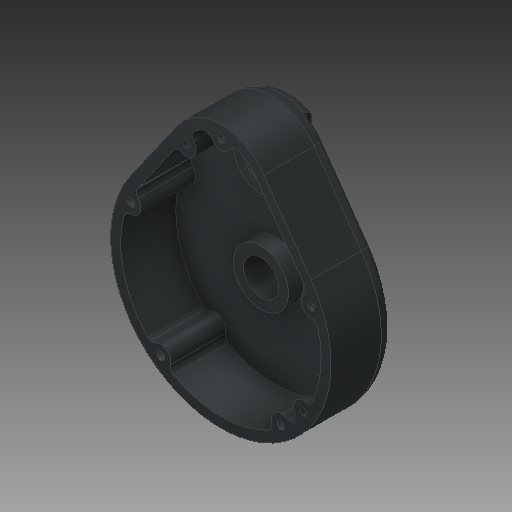
# Autodesk Inventor part: Caja1
Saved by Autodesk Inventor 2020 (Build 240168000, 168)
## iProperties
Created: 2016-04-19
Part Number: Caja1
Material: Iron, Cast
Document SubType Name: Modeling
Designer: Jorge
Density: 7.15 g/cm^3
Appearance: Iron Gray
Mass: 1669.68 g
Surface Area: 742.961 cm^2
Volume: 233.522 cm^3
Author: Jorge
Autodesk Inventor part; units mm, degrees
ref_plane "YZ Plane" through (0, 0, 0) normal (1, 0, 0) x (0, 1, 0)
ref_plane "XZ Plane" through (0, 0, 0) normal (0, 1, 0) x (-1, 0, 0)
ref_plane "XY Plane" through (0, 0, 0) normal (0, 0, 1) x (1, 0, 0)
sketch "Sketch1" plane through (0, 0, 0) normal (0, 0, 1) x (1, 0, 0)
  line L0 (57.148, 40.1638) -> (27.2752, 82.6691)
  arc A0 (27.2752, 82.6691) -> (-27.2752, 82.6691) centre (0, 63.5) ccw
  line L1 (-27.2752, 82.6691) -> (-57.148, 40.1638)
  arc A1 (-57.148, 40.1638) -> (57.148, 40.1638) centre (0, 0) ccw
  line L2 (-97.79, 0) -> (97.79, 0) construction
  circle A2 centre (0, 0) radius 11.1125
  circle A3 centre (0, 63.5) radius 11.1125
  line L3 (0, -103.1875) -> (0, 130.175) construction
  dimension "d21" = 33.3375
  dimension "d23" = 69.85
  dimension "d24" = 63.5
  dimension "d25" = 22.225
  dimension "d27" = 0
  constraints: 4 centre point, 4 end point, 4 point on circle, 4 tangent, 3 coincident, 1 equal radius
  measures "d21" radius of A0
  measures "d23" radius of A1
  measures "d24" distance of point (0, 0) A0.centre
  measures "d25" diameter of A2
  measures "d27" distance from line of L3 A0.centre
extrude "Extrusion2" add sketch "Sketch1" against normal blind 41.275
sketch "Sketch3" plane through (0, 0, 0) normal (0, 0, 1) x (1, 0, 0)
  circle A0 centre (0, 63.5) radius 11.1125 construction
  line L0 (-51.9527, 36.5125) -> (-29.9545, 67.8132)
  line L1 (22.0799, 79.0178) -> (51.9527, 36.5125)
  arc A1 (-57.4985, 19.0596) -> (-52.6772, 29.9074) centre (-57.15, 25.4) ccw
  arc A2 (-25.0533, 68.989) -> (-17.4133, 78.9063) centre (-22.0799, 74.5998) ccw
  arc A3 (-5.5475, 85.81) -> (5.5475, 85.81) centre (0, 88.9) ccw
  arc A4 (-32.0833, -51.2429) -> (-41.5727, -43.8962) centre (-38.1, -49.2125) ccw
  arc A5 (53.5354, -28.682) -> (47.0078, -38.3187) centre (52.3748, -34.925) ccw
  line L2 (0, -103.1875) -> (0, 130.175) construction
  line L3 (-97.79, 0) -> (97.79, 0) construction
  arc A6 (-51.9527, 36.5125) -> (-53.1847, 34.6935) centre (0, 0) ccw
  arc A7 (-61.3911, 16.2291) -> (-46.4429, -43.3048) centre (0, 0) ccw
  arc A8 (52.6772, 29.9074) -> (57.4985, 19.0596) centre (57.15, 25.4) ccw
  arc A9 (41.489, -43.8425) -> (32.0833, -51.2429) centre (38.1, -49.2125) ccw
  arc A10 (57.6934, -26.5278) -> (61.3911, 16.2291) centre (0, 0) ccw
  arc A11 (53.1847, 34.6935) -> (51.9527, 36.5125) centre (0, 0) ccw
  arc A12 (22.0799, 79.0178) -> (11.7884, 87.7767) centre (0, 63.5) ccw
  arc A13 (-11.7884, 87.7767) -> (-17.0156, 84.4474) centre (0, 63.5) ccw
  arc A14 (-25.0533, 68.989) -> (-29.9545, 67.8132) centre (-26.8374, 65.6225) ccw
  arc A15 (-53.1847, 34.6935) -> (-52.6772, 29.9074) centre (-49.9936, 32.6119) ccw
  arc A16 (-57.4985, 19.0596) -> (-61.3911, 16.2291) centre (-57.7076, 15.2553) ccw
  arc A17 (-46.4429, -43.3048) -> (-41.5727, -43.8962) centre (-43.6564, -40.7065) ccw
  arc A18 (-32.0833, -51.2429) -> (-30.2908, -55.8097) centre (-28.4734, -52.4611) ccw
  arc A19 (30.2908, -55.8097) -> (32.0833, -51.2429) centre (28.4734, -52.4611) ccw
  arc A20 (53.5354, -28.682) -> (57.6934, -26.5278) centre (54.2318, -24.9361) ccw
  arc A21 (61.3911, 16.2291) -> (57.4985, 19.0596) centre (57.7076, 15.2553) ccw
  arc A22 (52.6772, 29.9074) -> (53.1847, 34.6935) centre (49.9936, 32.6119) ccw
  arc A23 (-17.0156, 84.4474) -> (-17.4133, 78.9063) centre (-14.6134, 81.4901) ccw
  arc A24 (-5.5475, 85.81) -> (-11.7884, 87.7767) centre (-9.7081, 83.4926) ccw
  arc A25 (11.7884, 87.7767) -> (5.5475, 85.81) centre (9.7081, 83.4926) ccw
  arc A26 (41.489, -43.8425) -> (47.0078, -38.3187) centre (43.625, -40.4578) ccw
  arc A27 (-30.2908, -55.8097) -> (30.2908, -55.8097) centre (0, 0) ccw
  point P0 (-27.5047, 71.2991)
  dimension "d34" = 49.2125
  dimension "d35" = 25.4
  dimension "d36" = 57.15
  dimension "d37" = 38.1
  dimension "d38" = 74.5998
  dimension "d39" = 88.9
  dimension "d40" = 0
  dimension "d41" = 52.3748
  dimension "d42" = 34.925
  dimension "d43" = 6.35
  dimension "d45" = 26.9875
  dimension "d46" = 3.81
  dimension "d47" = 4.7625
  dimension "d111" = 4.0023
  constraints: 55 point on circle, 28 tangent, 27 centre point, 13 equal radius, 4 end point, 2 coincident, 2 symmetric about line, 1 point on line, 2 other
  measures "d34" distance from line of A4.centre L3
  measures "d35" distance from line of A1.centre L3
  measures "d36" distance from line of L2 A1.centre
  measures "d37" distance from line of L2 A4.centre
  measures "d38" distance from line of A2.centre L3
  measures "d39" distance from line of L3 A3.centre
  measures "d40" distance from line of L2 A3.centre
  measures "d41" distance from line of A5.centre L2
  measures "d42" distance from line of A5.centre L3
  measures "d43" radius of A3
  measures "d45" radius of A13
  measures "d46" radius of A14
  measures "d47" radius of A24
  measures "d111" radius of A26
extrude "Extrusion3" cut sketch "Sketch3" against normal blind 34.925
sketch "Sketch4" plane through (0, 0, -34.925) normal (0, 0, 1) x (1, 0, 0)
  circle A0 centre (0, 63.5) radius 11.1125 projected
  circle A1 centre (0, 0) radius 11.1125 projected
  arc A2 (-7.6278, 79.2085) -> (7.6278, 79.2085) centre (0, 63.5) ccw
  circle A3 centre (0, 0) radius 17.4625
  arc A4 (-5.5475, 85.81) -> (5.5475, 85.81) centre (0, 88.9) ccw projected
  arc A5 (-5.5475, 85.81) -> (5.5475, 85.81) centre (0, 88.9) ccw
  arc A6 (-7.6278, 79.2085) -> (-5.5475, 85.81) centre (-9.7081, 83.4926) ccw
  arc A7 (5.5475, 85.81) -> (7.6278, 79.2085) centre (9.7081, 83.4926) ccw
  arc A8 (-5.5475, 85.81) -> (5.5475, 85.81) centre (0, 88.9) ccw projected
  dimension "d48" = 34.925
  dimension "d51" = 4.7625
  constraints: 10 point on circle, 5 centre point, 4 tangent, 2 coincident, 2 equal radius, 1 concentric
  measures "d48" diameter of A3
  measures "d51" radius of A6
extrude "Extrusion4" add sketch "Sketch4" along normal blind 9.5631
sketch "Sketch7" plane through (0, 0, 0) normal (0, 1, 0) x (-1, 0, 0)
  line L0 (14.2875, -41.275) -> (-14.2875, -41.275)
  line L1 (-14.2875, -41.275) -> (-14.2875, -42.8625)
  line L2 (14.2875, -42.8625) -> (14.2875, -41.275)
  line L3 (0, -53.7345) -> (0, 8.9558) construction
  line L4 (-27.2752, -41.275) -> (27.2752, -41.275) construction
  arc A0 (7.9375, -44.45) -> (6.35, -44.45) centre (7.1438, -44.45) ccw
  line L5 (7.9375, -44.45) -> (12.7, -44.45)
  arc A1 (0, -44.45) -> (-1.5875, -44.45) centre (-0.7937, -44.45) ccw
  arc A2 (-7.9375, -44.45) -> (-9.525, -44.45) centre (-8.7312, -44.45) ccw
  line L6 (0, -44.45) -> (6.35, -44.45)
  line L7 (-12.7, -44.45) -> (-9.525, -44.45)
  line L8 (-7.9375, -44.45) -> (-1.5875, -44.45)
  arc A3 (-14.2875, -42.8625) -> (-12.7, -44.45) centre (-12.7, -42.8625) ccw
  arc A4 (12.7, -44.45) -> (14.2875, -42.8625) centre (12.7, -42.8625) ccw
  point P0 (0, 0)
  point P1 (-14.2875, -44.45)
  point P2 (14.2875, -44.45)
  dimension "d66" = 28.575
  dimension "d67" = 14.2875
  dimension "d69" = 0
  dimension "d70" = 7.1437
  dimension "d71" = 0.7937
  dimension "d74" = 7.9375
  dimension "d96" = 1.5875
  constraints: 14 end point, 10 point on circle, 5 centre point, 5 parallel, 4 point on line, 4 tangent, 2 horizontal, 1 equal radius, 1 perpendicular, 8 other
  measures "d66" distance between parallel lines of L1 L2
  measures "d67" distance between parallel lines of L3 L2
  measures "d69" distance between parallel lines of L4 L0
  measures "d70" distance from line of A0.centre L2
  measures "d71" radius of A0
  measures "d74" distance of A0.centre A1.centre
  measures "d96" radius of A3
extrude "Extrusion5" add sketch "Sketch7" along normal blind 96.8502 and the other way blind 69.85
sketch "Sketch8" plane through (0, 0, 0) normal (1, 0, 0) x (0, 1, 0)
  line L0 (0, -54.3176) -> (0, 9.0529) construction
  line L1 (40.1637, -41.275) -> (40.1637, -41.275) construction
  line L2 (96.8502, -43.6563) -> (-69.85, -43.6563) construction
  line L3 (-66.675, -41.275) -> (-78.3505, -41.275)
  line L4 (-69.85, -41.275) -> (-68.3732, -41.275) projected
  line L5 (-66.675, -41.275) -> (-66.675, -42.8625) construction
  line L6 (-78.3505, -41.275) -> (-78.3505, -44.5144)
  line L7 (-78.3505, -44.5144) -> (-61.1391, -44.5144)
  arc A0 (-66.675, -41.275) -> (-61.1391, -44.5144) centre (-61.1391, -38.1644) ccw
  point P0 (0, 0)
  point P1 (-65.0868, -44.5144)
  dimension "d84" = 0
  dimension "d87" = 66.675
  dimension "d106" = 6.35
  dimension "d107" = 3.2394
  constraints: 8 end point, 2 horizontal, 2 point on circle, 2 vertical, 1 centre point, 1 horizontal alignment, 1 point on line, 1 tangent
  measures "d84" distance between parallel lines of L4 L3
  measures "d87" distance between parallel lines of L5 L0
  measures "d106" radius of A0
  measures "d107" distance between parallel lines of L3 L7
revolve "Revolution1" cut sketch "Sketch8" angle 180 mid plane about axis through (0, 0, -10) along (0, 0, 1)
sketch "Sketch9" plane through (0, 0, 0) normal (1, 0, 0) x (0, 1, 0)
  line L0 (96.8502, -43.6563) -> (-63.7315, -43.6563) construction
  line L1 (93.6207, -41.275) -> (96.8502, -41.275) construction
  line L2 (82.6691, -41.275) -> (82.6691, -41.275) construction
  line L3 (93.6625, -41.275) -> (109.3342, -41.275)
  line L4 (63.5, 9.0374) -> (63.5, -54.2241) construction
  line L5 (109.3342, -44.45) -> (88.1632, -44.45)
  line L6 (93.6625, -41.275) -> (93.6625, -42.8625) construction
  line L7 (109.3342, -44.45) -> (109.3342, -41.275)
  arc A0 (88.1632, -44.45) -> (93.6625, -41.275) centre (88.1632, -38.1) ccw
  point P0 (0, 0)
  point P1 (92.075, -44.45)
  dimension "d98" = 30.1625
  dimension "d108" = 6.35
  dimension "d109" = 3.175
  constraints: 8 end point, 2 point on circle, 2 vertical, 1 centre point, 1 horizontal, 1 horizontal alignment, 1 parallel, 1 point on line, 1 tangent
  measures "d98" distance between parallel lines of L6 L4
  measures "d108" radius of A0
  measures "d109" distance from line of L3 L5.start
revolve "Revolution2" cut sketch "Sketch9" angle 90 mid plane about axis through (0, 63.5, 0) along (0, 0, -1)
sketch "Sketch10" plane through (0, 0, 0) normal (1, 0, 0) x (0, 1, 0)
  line L0 (-69.85, -44.45) -> (96.8502, -44.45) projected
  line L1 (-69.85, -41.275) -> (40.1638, -41.275) construction
  line L2 (-14.2875, -41.275) -> (-14.2875, -41.275)
  line L3 (0, -63.0631) -> (0, 10.5105) construction
  line L4 (-14.2875, -41.275) -> (0, -41.275)
  line L5 (11.1125, -41.275) -> (-11.1125, -41.275) projected
  line L6 (-19.7868, -44.45) -> (0, -44.45)
  line L7 (-69.85, -44.45) -> (96.8502, -44.45) projected
  line L8 (0, -44.45) -> (0, -41.275)
  line L9 (-69.85, -44.45) -> (96.8502, -44.45) projected
  arc A0 (-19.7868, -44.45) -> (-14.2875, -41.275) centre (-19.7868, -38.1) ccw
  line L10 (-14.2875, -41.275) -> (-14.2875, -52.5526) construction
  point P0 (0, 0)
  point P1 (-11.2175, -44.45)
  point P2 (-64.601, -44.45)
  point P3 (90.9504, -44.45)
  point P4 (-15.875, -44.45)
  point P5 (149.2752, -44.45)
  point P6 (-63.8357, -44.45)
  point P7 (89.0977, -44.45)
  point P8 (-61.531, -44.45)
  point P9 (-60.7271, -44.45)
  point P10 (84.642, -44.45)
  dimension "d103" = 6.35
  dimension "d104" = 14.2875
  constraints: 10 end point, 4 point on line, 2 point on circle, 1 centre point, 1 midpoint, 1 perpendicular, 1 tangent, 1 vertical, 3 other
  measures "d103" radius of A0
  measures "d104" distance between parallel lines of L3 L10
revolve "Revolution3" cut sketch "Sketch10" angle 360 about axis through (0, 0, -10) along (0, 0, 1)
sketch "Sketch11" plane through (0, 0, 0) normal (1, 0, 0) x (0, 1, 0)
  line L0 (-69.85, -44.45) -> (96.8502, -44.45) construction
  line L1 (82.6691, -41.275) -> (40.1638, -41.275) construction
  line L2 (63.5, -44.45) -> (83.2868, -44.45)
  line L3 (93.6207, -41.275) -> (-68.3732, -41.275) construction
  line L4 (63.5, -41.275) -> (77.7875, -41.275)
  line L5 (63.5, 9.0374) -> (63.5, -54.2241) construction
  line L6 (77.7875, -41.275) -> (77.7875, -42.8625) construction
  line L7 (63.5, -41.275) -> (63.5, -44.45)
  arc A0 (77.7875, -41.275) -> (83.2868, -44.45) centre (83.2868, -38.1) ccw
  line L8 (-69.85, -44.45) -> (96.8502, -44.45) projected
  point P0 (0, 0)
  point P1 (9.525, -44.45)
  point P2 (89.0977, -44.45)
  point P3 (53.0291, -44.45)
  point P4 (112.7637, -44.45)
  point P5 (90.064, -41.275)
  point P6 (0, -41.275)
  point P7 (-63.8357, -44.45)
  point P8 (15.1732, -44.45)
  point P9 (-65.1262, -41.275)
  point P10 (-60.7271, -44.45)
  point P11 (-15.1732, -44.45)
  dimension "d100" = 14.2875
  dimension "d105" = 6.35
  constraints: 8 end point, 5 point on line, 2 point on circle, 1 centre point, 1 collinear, 1 tangent, 1 vertical, 2 other
  measures "d100" distance between parallel lines of L5 L6
  measures "d105" radius of A0
revolve "Revolution4" cut sketch "Sketch11" angle 360 about axis through (0, 63.5, 0) along (0, 0, -1)
sketch "Sketch5" plane through (0, 0, 0) normal (0, 0, 1) x (1, 0, 0)
  arc A0 (-5.5475, 85.81) -> (5.5475, 85.81) centre (0, 88.9) ccw construction
  arc A1 (-57.4985, 19.0596) -> (-52.6772, 29.9074) centre (-57.15, 25.4) ccw construction
  arc A2 (-32.0833, -51.2429) -> (-41.5727, -43.8962) centre (-38.1, -49.2125) ccw construction
  arc A3 (53.5354, -28.682) -> (47.0078, -38.3187) centre (52.3748, -34.925) ccw construction
  arc A4 (52.6772, 29.9074) -> (57.4985, 19.0596) centre (57.15, 25.4) ccw construction
  point P0 (0, 0)
  point P1 (38.1, -49.2125)
  point P2 (47.0576, -38.3963)
  point P3 (38.1, -49.2125)
  constraints: 5 coincident
hole "Hole1" at (0, 88.9, 0) at (-57.15, 25.4, 0) at (-38.1, -49.2125, 0) at (38.1, -49.2125, 0) at (57.15, 25.4, 0) direction (0, 0, -1) diameter 4.9784 depth 15.875 tip angle 118 thread size "1/4-20 UNC" class "2B" standard "ANSI Unified Screw Threads"
sketch "Sketch6" plane through (0, 0, 0) normal (0, 0, 1) x (1, 0, 0)
  arc A0 (-25.0533, 68.989) -> (-17.4133, 78.9063) centre (-22.0799, 74.5998) ccw construction
  arc A1 (53.5354, -28.682) -> (47.0078, -38.3187) centre (52.3748, -34.925) ccw construction
  point P0 (0, 0)
  point P1 (47.0576, -38.3963)
hole "Hole2" at (-22.0799, 74.5998, 0) at (52.3748, -34.925, 0) direction (0, 0, -1) diameter 4.3688 depth 34.925 tip angle 118
fillet "Fillet1" radius 9.525 4 edges at (0, -69.85, -41.275) (-42.2116, 61.4164, -41.275) (0, 96.8375, -41.275) (42.2116, 61.4164, -41.275)
equation "\"d67\" = 0.5 * d66"
body "Solid2"
